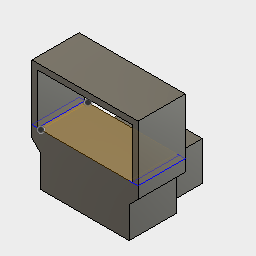
XT60 Mount v2 (Autodesk Fusion 360 design; units mm, degrees)
Autodesk Fusion 360 part; units mm, degrees
sketch "Sketch1" plane through (0, 0, 0) normal (0, 0, 1) x (1, 0, 0)
  line L0 (0, 0) -> (10.6, 0)
  line L1 (10.6, 0) -> (10.6, 6.6)
  line L2 (10.6, 6.6) -> (0, 6.6)
  line L3 (0, 6.6) -> (0, 0)
  dimension "d1" = 6.6
  dimension "d2" = 10.6
  constraint horizontal L0
  constraint vertical L1
  constraint horizontal L2
  constraint vertical L3
  constraint coincident L0.start L3.end
extrude "Extrude1" add sketch "Sketch1" along normal blind 6.6
sketch "Sketch2" plane through (0, 0, 6.6) normal (0, 0, 1) x (1, 0, 0)
  line L0 (0, 6.6) -> (0, 0)
  line L1 (0, 0) -> (10.6, 0)
  line L2 (10.6, 0) -> (10.6, 6.6)
  line L3 (10.6, 6.6) -> (0, 6.6)
  line L4 (0, 0) -> (-2.2, 0)
  line L5 (10.6, 0) -> (12.8, 0)
  line L6 (12.8, 0) -> (12.8, 8.8)
  line L7 (12.8, 8.8) -> (-2.2, 8.8)
  line L8 (-2.2, 8.8) -> (-2.2, 0)
  constraint coincident L0.end L1.start
  constraint parallel L2 L6
  constraint parallel L3 L7
  constraint parallel L0 L8
extrude "Extrude2" add sketch "Sketch2" along normal blind 8
sketch "Sketch3" plane through (0, 8.8, 0) normal (0, 1, 0) x (-1, 0, 0)
  line L0 (-12.8, 6.6) -> (2.2, 6.6)
  line L1 (2.2, 6.6) -> (2.2, 14.6)
  line L2 (2.2, 14.6) -> (-12.8, 14.6)
  line L3 (-12.8, 14.6) -> (-12.8, 6.6)
  line L4 (2.2, 14.6) -> (3.7, 14.6)
  line L5 (3.7, 14.6) -> (3.7, 6.6)
  line L6 (3.7, 6.6) -> (2.2, 6.6)
  line L7 (-12.8, 14.6) -> (-14.3, 14.6)
  line L8 (-14.3, 14.6) -> (-14.3, 6.6)
  line L9 (-14.3, 6.6) -> (-12.8, 6.6)
  line L10 (2.2, 6.6) -> (2.7, 6.6)
  line L11 (2.7, 6.6) -> (2.7, 14.6)
  line L12 (-12.8, 14.6) -> (-13.3, 14.6)
  line L13 (-13.3, 14.6) -> (-13.3, 6.6)
  line L14 (-13.3, 6.6) -> (-12.8, 6.6)
  dimension "d8" = 1.5
  dimension "d12" = 0.5
  dimension "d13" = 0.5
  constraint horizontal L4
  constraint perpendicular L0 L5
  constraint perpendicular L1 L6
  constraint perpendicular L5 L10
  constraint coincident L4
  constraint perpendicular L4 L11
  constraint perpendicular L3 L12
  constraint coincident L9 origin
  constraint perpendicular L9 L13
  constraint perpendicular L3 L14
extrude "Extrude4" add sketch "Sketch3" against normal blind 2 contours L3 L7 L9 L12 L13 L14 | L1 L4 L6 L10 L11
extrude "Extrude5" add sketch "Sketch3" along normal blind 9.5 and the other way blind 2 contours L7 L8 L9 L13 | L4 L5 L6 L11
sketch "Sketch5" plane through (-2.7, 0, 0) normal (1, 0, 0) x (0, 0, -1)
  line L0 (-14.6, 8.8) -> (-6.6, 8.8)
  line L1 (-6.6, 8.8) -> (-6.6, 18.3)
  line L2 (-6.6, 18.3) -> (-14.6, 18.3)
  line L3 (-14.6, 18.3) -> (-14.6, 8.8)
  line L4 (-14.6, 18.3) -> (-6.6, 18.3)
  line L5 (-6.6, 18.3) -> (-6.6, 17.3)
  line L6 (-6.6, 17.3) -> (-14.6, 17.3)
  line L7 (-14.6, 17.3) -> (-14.6, 18.3)
  dimension "d19" = 1
  dimension "d20" = 8
  constraint horizontal L4
  constraint vertical L5
  constraint horizontal L6
  constraint vertical L7
  measures "d19" distance of origin
extrude "Extrude6" add sketch "Sketch5" along normal blind 16 contours L1 L2 L3 L4 L5 L6 L7
chamfer "Chamfer1" distance 1.5 angle 45 2 edges at (-2.2, 6.8, 10.6) (12.8, 6.8, 10.6)
